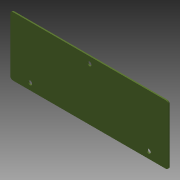
# Autodesk Inventor part: Veroboard
Saved by Autodesk Inventor 2015 (Build 190159000, 159)
## iProperties
Created: 2016-02-19
Part Number: Veroboard
Material: Generic
Document SubType Name: Modeling
Designer: 23902
Density: 1 g/cm^3
Appearance: Default
Author: 23902
Autodesk Inventor part; units mm, degrees
ref_plane "YZ Plane" through (0, 0, 0) normal (1, 0, 0) x (0, 1, 0)
ref_plane "XZ Plane" through (0, 0, 0) normal (0, 1, 0) x (-1, 0, 0)
ref_plane "XY Plane" through (0, 0, 0) normal (0, 0, 1) x (1, 0, 0)
sketch "Sketch1" plane through (0, 0, 0) normal (0, 1, 0) x (-1, 0, 0)
  circle A0 centre (-2.5953, 16.0933) radius 1.6
  circle A1 centre (-47.5953, -18.9067) radius 1.6
  line L0 (-47.5953, -23.9067) -> (55.4047, -23.9067)
  line L1 (-47.5953, -23.9067) -> (-60.5953, -23.9067)
  line L2 (-62.5953, -21.9067) -> (-62.5953, 19.0933)
  arc A2 (-62.5953, -21.9067) -> (-60.5953, -23.9067) centre (-60.5953, -21.9067) ccw
  line L3 (-60.5953, 21.0933) -> (55.4047, 21.0933)
  arc A3 (-60.5953, 21.0933) -> (-62.5953, 19.0933) centre (-60.5953, 19.0933) ccw
  line L4 (57.4047, 19.0933) -> (57.4047, -21.9067)
  arc A4 (57.4047, 19.0933) -> (55.4047, 21.0933) centre (55.4047, 19.0933) ccw
  arc A5 (55.4047, -23.9067) -> (57.4047, -21.9067) centre (55.4047, -21.9067) ccw
  circle A6 centre (42.4047, -18.9067) radius 1.6
  point P0 (0, 0)
  constraints: 10 end point, 8 point on circle, 7 centre point
extrude "Extrusion1" add sketch "Sketch1" along normal blind 1
body "Solid1"
